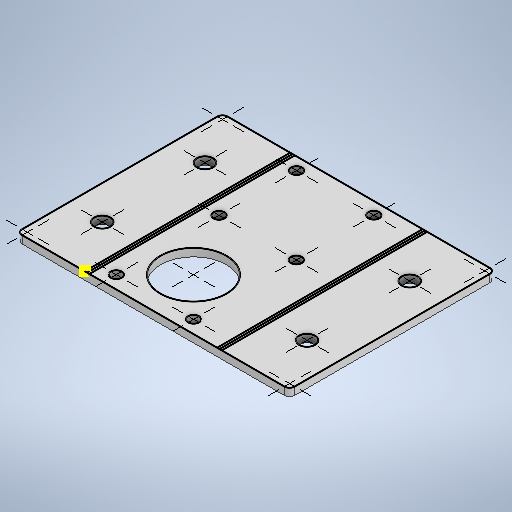
# Autodesk Inventor part: body_motor_L_frame
Saved by Autodesk Inventor 2026.1 (Build 301233000, 233)
## iProperties
Created: 2025-08-16
Part Number: body_motor_L_frame
Material: Generic
Document SubType Name: Modeling
Designer: chris
Density: 1 g/cm^3
Appearance: Default
Author: chris
Autodesk Inventor part; units mm, degrees
ref_plane "YZ Plane" through (0, 0, 0) normal (1, 0, 0) x (0, 1, 0)
ref_plane "XZ Plane" through (0, 0, 0) normal (0, 1, 0) x (-1, 0, 0)
ref_plane "XY Plane" through (0, 0, 0) normal (0, 0, 1) x (1, 0, 0)
sketch "Sketch1" plane through (0, 0, 0) normal (0, 1, 0) x (-1, 0, 0)
  line L0 (-26.2289, 0) -> (-26.2289, -40)
  line L1 (-0.4496, -40) -> (-0.4496, 0)
  circle A0 centre (6.595, -30) radius 1.55
  circle A1 centre (-33.2736, -30) radius 1.55
  circle A2 centre (6.595, -10) radius 1.55
  circle A3 centre (-33.2736, -10) radius 1.55
  circle A4 centre (-11.1593, -10) radius 6.4
  circle A5 centre (-3.6343, -2.5) radius 1.05
  circle A6 centre (-18.6843, -2.5) radius 1.05
  circle A7 centre (-18.6843, -22.5) radius 1.05
  circle A8 centre (-3.6343, -22.5) radius 1.05
  circle A9 centre (-3.6343, -37.6) radius 1.05
  circle A10 centre (-18.6843, -37.6) radius 1.05
  arc A11 (-38.8686, 0) -> (-39.8686, -1) centre (-38.8686, -1) ccw
  line L2 (-39.8686, -39) -> (-39.8686, -1)
  arc A12 (-39.8686, -39) -> (-38.8686, -40) centre (-38.8686, -39) ccw
  arc A13 (13.19, -1) -> (12.19, 0) centre (12.19, -1) ccw
  line L3 (-38.8686, 0) -> (12.19, 0)
  arc A14 (12.19, -40) -> (13.19, -39) centre (12.19, -39) ccw
  line L4 (12.19, -40) -> (-38.8686, -40)
  line L5 (13.19, -1) -> (13.19, -39)
  line L6 (-26.6786, -40) -> (-26.6786, 0)
  line L7 (-25.7793, 0) -> (-25.7793, -40)
  line L8 (-0.8993, -40) -> (-0.8993, 0)
  line L9 (0, 0) -> (0, -40)
  point P0 (0, 0)
  constraints: 20 end point, 15 centre point, 12 point on line, 11 equal radius, 8 point on circle, 8 tangent, 8 vertical, 7 parallel, 2 horizontal, 2 perpendicular, 51 other
extrude "Extrusion1" add sketch "Sketch1" against normal blind 1.5
body "Solid1"
